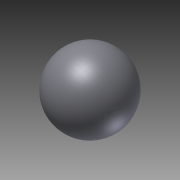
# Autodesk Inventor part: BallBearingBall
Saved by Autodesk Inventor 2012 SP1 (Build 160190100, 190)
## iProperties
Created: 2010-06-08
Part Number: BallBearingBall
Document SubType Name: Modeling
Designer: rconnaug
Density: 8.08 g/cm^3
Material: Stainless Steel
Mass: 0.703879 g
Surface Area: 0.950332 cm^2
Volume: 0.0871137 cm^3
Author: rconnaug
Autodesk Inventor part; units mm, degrees
ref_plane "YZ Plane" through (0, 0, 0) normal (1, 0, 0) x (0, 1, 0)
ref_plane "XZ Plane" through (0, 0, 0) normal (0, 1, 0) x (-1, 0, 0)
ref_plane "XY Plane" through (0, 0, 0) normal (0, 0, 1) x (1, 0, 0)
sketch "Sketch1" plane through (0, 0, 0) normal (0, 0, 1) x (1, 0, 0)
  arc A0 (0, -2.78) -> (0, 2.78) centre (0, 0) ccw
  line L0 (0, 2.78) -> (0, -11.0457)
  line L1 (-0.556, 0) -> (3.336, 0) projected
  line L2 (0, -13.8108) -> (0, 5.5451) projected
  dimension "d0" = 2.78
  constraints: 2 end point, 2 point on circle, 2 point on line, 1 centre point, 1 coincident, 1 collinear, 1 vertical
  measures "d0" radius of A0
revolve "Revolution1" add sketch "Sketch1" angle 360 about axis through (0, 2.78, 0) along (0, -1, 0)
body "Solid1"
